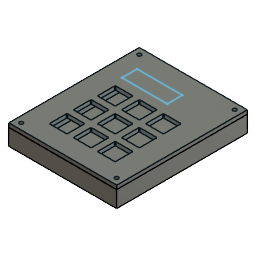
Dap-o-ram (FINAL) (Autodesk Fusion 360 archive; units mm, degrees)
design "Macropad (Hackclub)"
part number: 2026-06-12-01-53-34-415
Autodesk Fusion 360 part; units mm, degrees
derive "DerivedContext1"
sketch "Sketch1" plane through (0, 0, 0) normal (0, 1, 0) x (1, 0, 0)
  line L0 (-75.4, 93.4) -> (-10, 93.4)
  line L1 (-10, 93.4) -> (-10, 10)
  line L2 (-10, 10) -> (-75.4, 10)
  line L3 (-75.4, 10) -> (-75.4, 93.4)
  line L4 (-85.4, 103.4) -> (0, 103.4)
  line L5 (0, 103.4) -> (0, 0)
  line L6 (0, 0) -> (-85.4, 0)
  line L7 (-85.4, 0) -> (-85.4, 103.4)
  circle A0 centre (-80.4, 98.4) radius 1.45
  circle A1 centre (-5, 98.4) radius 1.45
  circle A2 centre (-5, 5) radius 1.45
  circle A3 centre (-80.4, 5) radius 1.45
  dimension "d1" = 65.4
  dimension "d2" = 83.4
  dimension "d3" = 85.4
  dimension "d4" = 103.4
  dimension "d10" = 2.9
  dimension "d11" = 2.9
  dimension "d12" = 2.9
  dimension "d13" = 2.9
  constraint horizontal L0
  constraint vertical L1
  constraint horizontal L2
  constraint vertical L3
  constraint horizontal L4
  constraint vertical L5
  constraint horizontal L6
  constraint vertical L7
  measures "d1" distance of L0.start L0.end
  measures "d2" distance of L0.start L2.end
  measures "d3" distance of L4.start L4.end
  measures "d4" distance of L4.start L6.end
  measures "d10" diameter of A0
  measures "d11" diameter of A1
  measures "d12" diameter of A2
  measures "d13" diameter of A3
extrude "Extrude1" add sketch "Sketch1" along normal blind 13 makes body 1
extrude "Extrude2" add sketch "Sketch1" along normal blind 3 contours L0 L1 L2 L3 bodies 1
sketch "Sketch9" plane through (0, 3, 0) normal (0, 1, 0) x (-1, 0, 0)
  line L0 (75.4, -10) -> (10, -10)
  line L1 (10, -10) -> (10, -93.4)
  line L2 (10, -93.4) -> (75.4, -93.4)
  line L3 (75.4, -93.4) -> (75.4, -10)
  line L4 (75.4, -50.0851) -> (71.2745, -50.0851)
  line L5 (62.1435, -93.4) -> (62.1435, -71.701)
  line L6 (46, -10) -> (46, -13)
  line L7 (75.4, -50.0851) -> (71.2745, -50.0851)
  line L8 (10, -50) -> (14.1255, -50)
  dimension "d22" = 4.1255
  dimension "d24" = 21.699
  dimension "d25" = 3
  dimension "d26" = 4.1255
  dimension "d27" = 4.1255
  constraint coincident L3 L4.start
  constraint perpendicular L3 L4
  constraint coincident L2 L5.start
  constraint perpendicular L2 L5
  constraint coincident L0 L6.start
  constraint perpendicular L0 L6
  constraint coincident L1 L8.start
  constraint perpendicular L1 L8
  measures "d22" distance of L4.start L4.end
  measures "d24" distance of L5.start L5.end
  measures "d25" distance of L6.start L6.end
  measures "d26" distance of L4.start L4.end
  measures "d27" distance of L8.start L8.end
sketch "Sketch10" plane through (0, 3, 0) normal (0, 1, 0) x (-1, 0, 0)
  line L0 (14.125, -70.15, 10) -> (71.275, -70.15, 10)
  line L1 (14.125, -13, 10) -> (71.275, -13, 10)
  line L2 (49.7, -35.075, 10) -> (49.7, -48.075, 10)
  line L3 (14.125, -70.15, 10) -> (14.125, -13, 10)
  line L4 (35.7, -54.125, 10) -> (35.7, -67.125, 10)
  line L5 (17.15, -34.575, 10) -> (30.15, -34.575, 10)
  line L6 (35.7, -35.075, 10) -> (35.7, -48.075, 10)
  line L7 (30.65, -16.025, 10) -> (30.65, -29.025, 10)
  arc A0 through (49.2, -48.575, 10) (49.5536, -48.4286, 10) (49.7, -48.075, 10)
  arc A1 through (30.65, -54.125, 10) (30.5036, -53.7714, 10) (30.15, -53.625, 10)
  arc A2 through (30.15, -48.575, 10) (30.5036, -48.4286, 10) (30.65, -48.075, 10)
  arc A3 through (16.65, -48.075, 10) (16.7964, -48.4286, 10) (17.15, -48.575, 10)
  line L8 (17.15, -53.625, 10) -> (30.15, -53.625, 10)
  arc A4 through (35.7, -67.125, 10) (35.8464, -67.4786, 10) (36.2, -67.625, 10)
  arc A5 through (16.65, -29.025, 10) (16.7964, -29.3786, 10) (17.15, -29.525, 10)
  arc A6 through (30.15, -67.625, 10) (30.5036, -67.4786, 10) (30.65, -67.125, 10)
  arc A7 through (49.2, -67.625, 10) (49.5536, -67.4786, 10) (49.7, -67.125, 10)
  line L9 (17.15, -29.525, 10) -> (30.15, -29.525, 10)
  line L10 (30.65, -54.125, 10) -> (30.65, -67.125, 10)
  arc A8 through (36.2, -34.575, 10) (35.8464, -34.7214, 10) (35.7, -35.075, 10)
  line L11 (17.15, -15.525, 10) -> (30.15, -15.525, 10)
  line L12 (36.2, -67.625, 10) -> (49.2, -67.625, 10)
  arc A9 through (35.7, -48.075, 10) (35.8464, -48.4286, 10) (36.2, -48.575, 10)
  line L13 (54.75, -54.125, 10) -> (54.75, -67.125, 10)
  line L14 (36.2, -48.575, 10) -> (49.2, -48.575, 10)
  line L15 (17.15, -48.575, 10) -> (30.15, -48.575, 10)
  arc A10 through (17.15, -15.525, 10) (16.7964, -15.6714, 10) (16.65, -16.025, 10)
  line L16 (49.7, -54.125, 10) -> (49.7, -67.125, 10)
  line L17 (16.65, -54.125, 10) -> (16.65, -67.125, 10)
  arc A11 through (54.75, -67.125, 10) (54.8964, -67.4786, 10) (55.25, -67.625, 10)
  arc A12 through (68.75, -54.125, 10) (68.6036, -53.7714, 10) (68.25, -53.625, 10)
  arc A13 through (68.25, -48.575, 10) (68.6036, -48.4286, 10) (68.75, -48.075, 10)
  arc A14 through (49.7, -16.025, 10) (49.5536, -15.6714, 10) (49.2, -15.525, 10)
  arc A15 through (68.75, -35.075, 10) (68.6036, -34.7214, 10) (68.25, -34.575, 10)
  line L18 (36.2, -29.525, 10) -> (49.2, -29.525, 10)
  arc A16 through (68.25, -29.525, 10) (68.6036, -29.3786, 10) (68.75, -29.025, 10)
  arc A17 through (35.7, -29.025, 10) (35.8464, -29.3786, 10) (36.2, -29.525, 10)
  arc A18 through (49.7, -35.075, 10) (49.5536, -34.7214, 10) (49.2, -34.575, 10)
  arc A19 through (49.2, -29.525, 10) (49.5536, -29.3786, 10) (49.7, -29.025, 10)
  line L19 (68.75, -35.075, 10) -> (68.75, -48.075, 10)
  arc A20 through (54.75, -29.025, 10) (54.8964, -29.3786, 10) (55.25, -29.525, 10)
  line L20 (55.25, -15.525, 10) -> (68.25, -15.525, 10)
  line L21 (55.25, -67.625, 10) -> (68.25, -67.625, 10)
  arc A21 through (49.7, -54.125, 10) (49.5536, -53.7714, 10) (49.2, -53.625, 10)
  arc A22 through (30.65, -35.075, 10) (30.5036, -34.7214, 10) (30.15, -34.575, 10)
  line L22 (68.75, -54.125, 10) -> (68.75, -67.125, 10)
  arc A23 through (36.2, -15.525, 10) (35.8464, -15.6714, 10) (35.7, -16.025, 10)
  line L23 (55.25, -34.575, 10) -> (68.25, -34.575, 10)
  line L24 (49.7, -16.025, 10) -> (49.7, -29.025, 10)
  line L25 (68.75, -16.025, 10) -> (68.75, -29.025, 10)
  arc A24 through (54.75, -48.075, 10) (54.8964, -48.4286, 10) (55.25, -48.575, 10)
  line L26 (55.25, -48.575, 10) -> (68.25, -48.575, 10)
  line L27 (36.2, -15.525, 10) -> (49.2, -15.525, 10)
  line L28 (30.65, -35.075, 10) -> (30.65, -48.075, 10)
  line L29 (16.65, -16.025, 10) -> (16.65, -29.025, 10)
  line L30 (36.2, -34.575, 10) -> (49.2, -34.575, 10)
  arc A25 through (16.65, -67.125, 10) (16.7964, -67.4786, 10) (17.15, -67.625, 10)
  arc A26 through (55.25, -53.625, 10) (54.8964, -53.7714, 10) (54.75, -54.125, 10)
  arc A27 through (17.15, -34.575, 10) (16.7964, -34.7214, 10) (16.65, -35.075, 10)
  line L31 (55.25, -53.625, 10) -> (68.25, -53.625, 10)
  arc A28 through (30.15, -29.525, 10) (30.5036, -29.3786, 10) (30.65, -29.025, 10)
  arc A29 through (17.15, -53.625, 10) (16.7964, -53.7714, 10) (16.65, -54.125, 10)
  arc A30 through (36.2, -53.625, 10) (35.8464, -53.7714, 10) (35.7, -54.125, 10)
  line L32 (17.15, -67.625, 10) -> (30.15, -67.625, 10)
  line L33 (16.65, -35.075, 10) -> (16.65, -48.075, 10)
  arc A31 through (68.25, -67.625, 10) (68.6036, -67.4786, 10) (68.75, -67.125, 10)
  line L34 (54.75, -35.075, 10) -> (54.75, -48.075, 10)
  line L35 (54.75, -16.025, 10) -> (54.75, -29.025, 10)
  arc A32 through (68.75, -16.025, 10) (68.6036, -15.6714, 10) (68.25, -15.525, 10)
  arc A33 through (55.25, -34.575, 10) (54.8964, -34.7214, 10) (54.75, -35.075, 10)
  arc A34 through (55.25, -15.525, 10) (54.8964, -15.6714, 10) (54.75, -16.025, 10)
  arc A35 through (30.65, -16.025, 10) (30.5036, -15.6714, 10) (30.15, -15.525, 10)
  line L36 (35.7, -16.025, 10) -> (35.7, -29.025, 10)
  line L37 (55.25, -29.525, 10) -> (68.25, -29.525, 10)
  line L38 (36.2, -53.625, 10) -> (49.2, -53.625, 10)
  line L39 (71.275, -70.15, 10) -> (71.275, -13, 10)
extrude "Extrude3" add sketch "Sketch10" along normal blind 3 separate body contours L0 L1 L3 L39 in plane through (0, 13, 0) normal (0, 1, 0) makes body 2
extrude "Extrude4" add 1 faces at (-14.125, 14, -51.1) along direction (1, 0, 0) blind 14.1255 on bodies 2 bodies 1 2
extrude "Extrude5" add 1 faces at (-71.275, 14, -51.1) along direction (-1, 0, 0) blind 14.1255 on bodies 1 bodies 1
extrude "Extrude6" add 1 faces at (-53.6, 15, -13) along direction (0, 0, 1) blind 12.9 on bodies 1 bodies 1
extrude "Extrude7" cut sketch "Sketch1" along normal blind 20 contours A3 bodies 1
extrude "Extrude8" cut 1 faces at (-5.3343, 13, -5.5962) along direction (0, 1, 0) blind 3 on bodies 1 bodies 1
sketch "Sketch12" plane through (0, 0, -93.4) normal (0, 0, 1) x (1, 0, 0)
  line L0 (-75.4, 3) -> (-10, 3)
  line L1 (-10, 3) -> (-10, 13)
  line L2 (-10, 13) -> (-75.4, 13)
  line L3 (-75.4, 13) -> (-75.4, 3)
  line L4 (-75.4, 8) -> (-47.601, 8)
  line L5 (-10, 8) -> (-38.184, 8)
  line L6 (-47.601, 8) -> (-47.601, 7.6)
  line L7 (-43, 3) -> (-43, 6.5)
  line L8 (-46.601, 9.3) -> (-39.184, 9.3)
  arc A0 (-47.601, 7.5) -> (-46.601, 6.5) centre (-46.601, 7.5) ccw
  line L9 (-38.184, 8.3) -> (-38.184, 7.9)
  arc A1 (-39.184, 6.5) -> (-38.184, 7.5) centre (-39.184, 7.5) ccw
  line L10 (-39.184, 6.5) -> (-46.601, 6.5)
  line L11 (-38.184, 8.3) -> (-38.184, 7.5)
  arc A2 (-38.184, 8.3) -> (-39.184, 9.3) centre (-39.184, 8.3) ccw
  arc A3 (-46.601, 9.3) -> (-47.601, 8.3) centre (-46.601, 8.3) ccw
  line L12 (-47.601, 7.9) -> (-47.601, 7.5)
  line L13 (-47.601, 8.3) -> (-47.601, 8)
  point P0 (-43, 6.4)
  dimension "d40" = 27.799
  dimension "d41" = 28.184
  dimension "d49" = 3.5
  dimension "d52" = 1
  dimension "d53" = 1
  dimension "d54" = 1
  dimension "d55" = 1
  constraint midpoint L3 L4.start
  constraint perpendicular L3 L4
  constraint midpoint L1 L5.start
  constraint perpendicular L1 L5
  constraint coincident L0 L7.start
  constraint perpendicular L0 L7
  constraint horizontal L8
  constraint vertical L11
  constraint horizontal L10
  constraint tangent L8 A3
  constraint tangent A1 L11
  constraint tangent A1 L10
  constraint tangent A0 L10
  constraint tangent L8 A2
  constraint tangent L11 A2
  constraint tangent A3 L13
  measures "d40" distance of L4.start L4.end
  measures "d41" distance of L5.start L5.end
  measures "d49" distance of L7.start L7.end
  measures "d52" radius of A3
  measures "d53" radius of A1
  measures "d54" radius of A0
  measures "d55" radius of A2
extrude "Extrude9" cut sketch "Sketch12" against normal blind 10 contours L6 L8 A0 L9 A1 L10 L11 A2 A3 L12 L13 bodies 1
extrude "Extrude10" add 1 faces at (-53.6, 15, -70.15) along direction (0, 0, -1) blind 33.2 on bodies 1 bodies 1
extrude "Extrude11" cut 1 faces at (-4.5911, 13, -98.9642) along direction (0, 1, 0) blind 3 on bodies 1 bodies 1
extrude "Extrude12" cut 1 faces at (-80.5076, 13, -99.5287) along direction (0, 1, 0) blind 3 on bodies 1 bodies 1
split "Split1" by plane through (-42.7, 13, -51.725) normal (0, 1, 0) bodies 1 makes body 3 at (-44.8667, 16, -88.3193)
sketch "Sketch14" plane through (0, 16, 0) normal (0, 1, 0) x (-1, 0, 0)
  circle A0 centre (5, -98.4) radius 1.45
  circle A1 centre (80.4, -5) radius 1.45
  line L0 (35.7, -48.075) -> (35.7, -35.075)
  arc A2 (36.2, -34.575) -> (35.7, -35.075) centre (36.2, -35.075) ccw
  line L1 (36.2, -34.575) -> (49.2, -34.575)
  arc A3 (49.7, -35.075) -> (49.2, -34.575) centre (49.2, -35.075) ccw
  line L2 (49.7, -35.075) -> (49.7, -48.075)
  arc A4 (49.2, -48.575) -> (49.7, -48.075) centre (49.2, -48.075) ccw
  line L3 (49.2, -48.575) -> (36.2, -48.575)
  arc A5 (35.7, -48.075) -> (36.2, -48.575) centre (36.2, -48.075) ccw
  arc A6 (68.75, -35.075) -> (68.25, -34.575) centre (68.25, -35.075) ccw
  line L4 (68.75, -35.075) -> (68.75, -48.075)
  arc A7 (68.25, -48.575) -> (68.75, -48.075) centre (68.25, -48.075) ccw
  line L5 (68.25, -48.575) -> (55.25, -48.575)
  arc A8 (54.75, -48.075) -> (55.25, -48.575) centre (55.25, -48.075) ccw
  line L6 (54.75, -48.075) -> (54.75, -35.075)
  arc A9 (55.25, -34.575) -> (54.75, -35.075) centre (55.25, -35.075) ccw
  line L7 (55.25, -34.575) -> (68.25, -34.575)
  line L8 (35.7, -67.125) -> (35.7, -54.125)
  arc A10 (36.2, -53.625) -> (35.7, -54.125) centre (36.2, -54.125) ccw
  line L9 (36.2, -53.625) -> (49.2, -53.625)
  arc A11 (49.7, -54.125) -> (49.2, -53.625) centre (49.2, -54.125) ccw
  line L10 (49.7, -54.125) -> (49.7, -67.125)
  arc A12 (49.2, -67.625) -> (49.7, -67.125) centre (49.2, -67.125) ccw
  line L11 (49.2, -67.625) -> (36.2, -67.625)
  arc A13 (35.7, -67.125) -> (36.2, -67.625) centre (36.2, -67.125) ccw
  arc A14 (55.25, -53.625) -> (54.75, -54.125) centre (55.25, -54.125) ccw
  line L12 (55.25, -53.625) -> (68.25, -53.625)
  arc A15 (68.75, -54.125) -> (68.25, -53.625) centre (68.25, -54.125) ccw
  line L13 (68.75, -54.125) -> (68.75, -67.125)
  arc A16 (68.25, -67.625) -> (68.75, -67.125) centre (68.25, -67.125) ccw
  line L14 (68.25, -67.625) -> (55.25, -67.625)
  arc A17 (54.75, -67.125) -> (55.25, -67.625) centre (55.25, -67.125) ccw
  line L15 (54.75, -67.125) -> (54.75, -54.125)
  arc A18 (17.15, -34.575) -> (16.65, -35.075) centre (17.15, -35.075) ccw
  line L16 (17.15, -34.575) -> (30.15, -34.575)
  arc A19 (30.65, -35.075) -> (30.15, -34.575) centre (30.15, -35.075) ccw
  line L17 (30.65, -35.075) -> (30.65, -48.075)
  arc A20 (30.15, -48.575) -> (30.65, -48.075) centre (30.15, -48.075) ccw
  line L18 (30.15, -48.575) -> (17.15, -48.575)
  arc A21 (16.65, -48.075) -> (17.15, -48.575) centre (17.15, -48.075) ccw
  line L19 (16.65, -48.075) -> (16.65, -35.075)
  arc A22 (36.2, -15.525) -> (35.7, -16.025) centre (36.2, -16.025) ccw
  line L20 (36.2, -15.525) -> (49.2, -15.525)
  arc A23 (49.7, -16.025) -> (49.2, -15.525) centre (49.2, -16.025) ccw
  line L21 (49.7, -16.025) -> (49.7, -29.025)
  arc A24 (49.2, -29.525) -> (49.7, -29.025) centre (49.2, -29.025) ccw
  line L22 (49.2, -29.525) -> (36.2, -29.525)
  arc A25 (35.7, -29.025) -> (36.2, -29.525) centre (36.2, -29.025) ccw
  line L23 (35.7, -29.025) -> (35.7, -16.025)
  arc A26 (17.15, -53.625) -> (16.65, -54.125) centre (17.15, -54.125) ccw
  line L24 (17.15, -53.625) -> (30.15, -53.625)
  arc A27 (30.65, -54.125) -> (30.15, -53.625) centre (30.15, -54.125) ccw
  line L25 (30.65, -54.125) -> (30.65, -67.125)
  arc A28 (30.15, -67.625) -> (30.65, -67.125) centre (30.15, -67.125) ccw
  line L26 (30.15, -67.625) -> (17.15, -67.625)
  arc A29 (16.65, -67.125) -> (17.15, -67.625) centre (17.15, -67.125) ccw
  line L27 (16.65, -67.125) -> (16.65, -54.125)
  arc A30 (55.25, -15.525) -> (54.75, -16.025) centre (55.25, -16.025) ccw
  line L28 (55.25, -15.525) -> (68.25, -15.525)
  arc A31 (68.75, -16.025) -> (68.25, -15.525) centre (68.25, -16.025) ccw
  line L29 (68.75, -16.025) -> (68.75, -29.025)
  arc A32 (68.25, -29.525) -> (68.75, -29.025) centre (68.25, -29.025) ccw
  line L30 (68.25, -29.525) -> (55.25, -29.525)
  arc A33 (54.75, -29.025) -> (55.25, -29.525) centre (55.25, -29.025) ccw
  line L31 (54.75, -29.025) -> (54.75, -16.025)
  line L32 (85.4005, -103.35) -> (85.4005, -0.1)
  line L33 (85.4005, -0.1) -> (-0.0005, -0.1)
  line L34 (-0.0005, -0.1) -> (-0.0005, -103.35)
  line L35 (-0.0005, -103.35) -> (85.4005, -103.35)
  arc A34 (17.15, -15.525) -> (16.65, -16.025) centre (17.15, -16.025) ccw
  line L36 (17.15, -15.525) -> (30.15, -15.525)
  arc A35 (30.65, -16.025) -> (30.15, -15.525) centre (30.15, -16.025) ccw
  line L37 (30.65, -16.025) -> (30.65, -29.025)
  arc A36 (30.15, -29.525) -> (30.65, -29.025) centre (30.15, -29.025) ccw
  line L38 (30.15, -29.525) -> (17.15, -29.525)
  arc A37 (16.65, -29.025) -> (17.15, -29.525) centre (17.15, -29.025) ccw
  line L39 (16.65, -29.025) -> (16.65, -16.025)
  circle A38 centre (5, -5) radius 1.45
  circle A39 centre (80.4, -98.4) radius 1.45
  line L40 (71.3781, -87.5967) -> (35.5781, -87.5967)
  line L41 (35.5781, -87.5967) -> (35.5781, -75.5967)
  line L42 (35.5781, -75.5967) -> (71.3781, -75.5967)
  line L43 (71.3781, -75.5967) -> (71.3781, -87.5967)
  dimension "d64" = 12
  dimension "d65" = 35.8
  constraint horizontal L40
  constraint vertical L41
  constraint horizontal L42
  constraint vertical L43
  measures "d64" distance of L40.start L42.end
  measures "d65" distance of L40.start L40.end
move_body "Move1" bodies 3 to x (1, 0, 0) y (0, 1, 0) z (0, 0, 1) at (0, 25, 0)
move_body "Move2" bodies 3 to x (1, 0, 0) y (0, 1, 0) z (0, 0, 1) at (0, -25, 0)
named bodies: "Bottom Case", "Top Lid"
